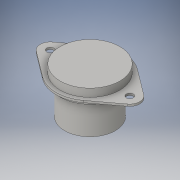
# Autodesk Inventor part: tube socket 9 pin
Saved by Autodesk Inventor 2016 (Build 200138000, 138)
## iProperties
Created: 2015-10-14
Part Number: tube socket 9 pin
Material: Generic
Document SubType Name: Modeling
Designer: jeremyhale
Density: 1 g/cm^3
Appearance: Default
Author: jeremyhale
Autodesk Inventor part; units mm, degrees
ref_plane "YZ Plane" through (0, 0, 0) normal (1, 0, 0) x (0, 1, 0)
ref_plane "XZ Plane" through (0, 0, 0) normal (0, 1, 0) x (-1, 0, 0)
ref_plane "XY Plane" through (0, 0, 0) normal (0, 0, 1) x (1, 0, 0)
sketch "Sketch1" plane through (0, 0, 0) normal (0, 1, 0) x (-1, 0, 0)
  line L0 (0, 0) -> (20, 0) construction
  circle A0 centre (20, 0) radius 1.75
  line L1 (0, 0) -> (25, 0) construction
  line L2 (25, 0) -> (25, -10) construction
  line L3 (10.2, 13.6) -> (23, 4)
  line L4 (10.2, -13.6) -> (23, -4)
  arc A1 (23, -4) -> (23, 4) centre (20, 0) ccw
  line L5 (0, 0) -> (0, -10)
  circle A2 centre (-20, 0) radius 1.75
  line L6 (-10.2, 13.6) -> (-23, 4)
  line L7 (-10.2, -13.6) -> (-23, -4)
  arc A3 (-23, 4) -> (-23, -4) centre (-20, 0) ccw
  arc A4 (10.2, 13.6) -> (-10.2, 13.6) centre (0, 0) ccw
  arc A5 (-10.2, -13.6) -> (10.2, -13.6) centre (0, 0) ccw
  dimension "d1" = 20
  dimension "d2" = 3.5
  dimension "d3" = 25
  dimension "d7" = 17
  dimension "d20" = 10
  dimension "d21" = 10
  constraints: 16 end point, 8 point on circle, 8 symmetric about line, 6 centre point, 4 coincident, 3 tangent, 2 horizontal, 2 vertical, 2 other
  measures "d1" distance of L0.start L0.end
  measures "d2" diameter of A0
  measures "d3" distance of L0.start L1.end
  measures "d7" radius of A4
  measures "d20" distance of L0.start L5.end
  measures "d21" distance of L1.end L2.end
extrude "Extrusion1" add sketch "Sketch1" along normal blind 1
sketch "Sketch2" plane through (0, 1, 0) normal (0, 1, 0) x (1, 0, 0)
  circle A0 centre (0, 0) radius 15
  dimension "d11" = 30
  constraints: 1 centre point, 1 coincident
  measures "d11" diameter of A0
extrude "Extrusion2" add sketch "Sketch2" along normal blind 4 and the other way blind 3
sketch "Sketch3" plane through (0, -2, 0) normal (0, -1, 0) x (1, 0, 0)
  circle A0 centre (0, 0) radius 12.7
  dimension "d15" = 25.4
  constraints: 1 centre point, 1 coincident
  measures "d15" diameter of A0
extrude "Extrusion3" add sketch "Sketch3" along normal blind 15.8
body "Solid1"
